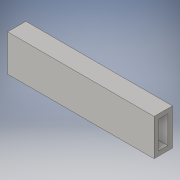
# Autodesk Inventor part: LiftSpacer
Saved by Autodesk Inventor 2016 SP1 (Build 200210100, 210)
## iProperties
Created: 2016-02-05
Part Number: LiftSpacer
Material: Generic
Document SubType Name: Modeling
Designer: steele
Density: 1 g/cm^3
Appearance: Default
Author: steele
Autodesk Inventor part; units mm, degrees
ref_plane "YZ Plane" through (0, 0, 0) normal (1, 0, 0) x (0, 1, 0)
ref_plane "XZ Plane" through (0, 0, 0) normal (0, 1, 0) x (-1, 0, 0)
ref_plane "XY Plane" through (0, 0, 0) normal (0, 0, 1) x (1, 0, 0)
sketch "Sketch1" plane through (0, 0, 0) normal (1, 0, 0) x (0, 1, 0)
  line L0 (-12.7, 6.35) -> (-12.7, -6.35)
  line L1 (-12.7, -6.35) -> (12.7, -6.35)
  line L2 (12.7, -6.35) -> (12.7, 6.35)
  line L3 (12.7, 6.35) -> (-12.7, 6.35)
  line L4 (-12.7, 6.35) -> (12.7, -6.35) construction
  line L5 (-12.7, -6.35) -> (12.7, 6.35) construction
  line L6 (-9.525, 3.175) -> (-9.525, -3.175)
  line L7 (-9.525, -3.175) -> (9.525, -3.175)
  line L8 (9.525, -3.175) -> (9.525, 3.175)
  line L9 (9.525, 3.175) -> (-9.525, 3.175)
  line L10 (-9.525, 3.175) -> (9.525, -3.175) construction
  line L11 (-9.525, -3.175) -> (9.525, 3.175) construction
  point P0 (0, 0)
  dimension "d0" = 12.7
  dimension "d1" = 25.4
  dimension "d4" = 3.175
  dimension "d5" = 3.175
  constraints: 24 end point, 4 midpoint, 4 parallel, 2 perpendicular, 2 vertical
  measures "d0" distance of L0.start L0.end
  measures "d1" distance of L2.end L0.start
  measures "d4" distance between parallel lines of L6 L0
  measures "d5" distance between parallel lines of L3 L9
extrude "Extrusion2" add sketch "Sketch1" along normal mid plane 101.6
body "Solid2"
